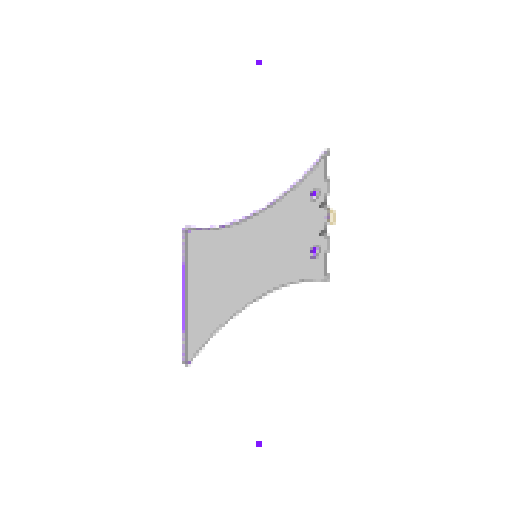
# Autodesk Inventor part: грань тела
Saved by Autodesk Inventor 2023.2 (Build 272271030, 271C)
## iProperties
Created: 2024-11-21
Part Number: грань тела
Material: Типовые
Document SubType Name: Modeling
Designer: DELL
Density: 1 g/cm^3
Appearance: По умолчанию
Author: DELL
Autodesk Inventor part; units mm, degrees
ref_plane "YZ Plane" through (0, 0, 0) normal (1, 0, 0) x (0, 1, 0)
ref_plane "XZ Plane" through (0, 0, 0) normal (0, 1, 0) x (-1, 0, 0)
ref_plane "РабПлоскость1" through (0, 0, -4) normal (0, 0, 1) x (1, 0, 0)
sketch "Эскиз10" plane through (0, 0, 0) normal (1, 0, 0) x (0, 1, 0)
  line L0 (-120, -3.999984) -> (120, -3.999996) construction
  line L1 (120, -3.999996) -> (120, 276.000004) construction
  line L2 (110.388959, 276.000004) -> (-110.388959, 276.000004)
  line L3 (-120, 276.000004) -> (-120, -3.999984) construction
  line L4 (-110, -3.999985) -> (110, -3.999996)
  arc A0 (-110, -3.999985) -> (-114.536812, 268.208047) centre (-321.93085, 128.609648) ccw
  arc A1 (114.536839, 268.208035) -> (110, -3.999996) centre (321.930876, 128.609584) ccw
  arc A2 (114.536839, 268.208035) -> (110.388959, 276.000004) centre (110.388986, 270.999993) ccw
  arc A3 (-110.388959, 276.000004) -> (-114.536812, 268.208047) centre (-110.388931, 271.000015) ccw
  ellipse E0 centre (-0.000042, -3.999995) end of major axis (-110.000042, -3.999985) minor radius 0.000001 (-77.388201, -3.999987) -> (77.387813, -4.000003) ccw
  point P0 (0, 0)
  point P1 (0, -3.999996)
  dimension "d55" = 5
  dimension "d50" = 240
  dimension "d51" = 280
  dimension "d52" = 220
  dimension "d53" = 250
  dimension "d54" = 250
  constraints: 10 end point, 6 point on circle, 4 horizontal, 2 centre point, 2 midpoint, 2 parallel, 2 point on line, 1 perpendicular, 12 other
  measures "d50" distance of L3.start L1.end
  measures "d51" distance of L1.end L0.end
  measures "d52" distance of L4.start L4.end
  measures "d53" radius of A0
  measures "d54" radius of A1
extrude "Выдавливание6" add sketch "Эскиз10" along normal mid plane 4
sketch "Эскиз12" plane through (2, 0, 0) normal (1, 0, 0) x (0, 0, -1)
  line L0 (4.106727, -100.959277) -> (0, -100.959277)
  line L1 (0, -100.959277) -> (0, -60.959277)
  line L2 (0, -60.959277) -> (3.999996, -60.959277)
  line L3 (3.999996, 110) -> (3.999996, -110)
  line L4 (3.999996, -110) -> (3.999996, 110)
  line L5 (3.999996, -35.959277) -> (0, -35.959277)
  line L6 (0, -35.959277) -> (0, -12.5)
  line L7 (0, -12.5) -> (3.999996, -12.5)
  line L8 (3.999996, 12.5) -> (0, 12.5)
  line L9 (0, 12.5) -> (0, 35.500352)
  line L10 (0, 35.500352) -> (3.999996, 35.500352)
  line L11 (3.999996, 60.500352) -> (0, 60.500352)
  line L12 (0, 60.500352) -> (0, 100.500352)
  line L13 (0, 100.500352) -> (3.999996, 100.500352)
  point P0 (0, 0)
  point P1 (3.999996, 12.5)
  point P2 (3.999996, 35.500352)
  point P3 (3.999996, -35.959277)
  point P4 (3.999996, -12.5)
  point P5 (3.999996, -100.959277)
  constraints: 24 end point, 10 perpendicular, 7 point on line, 2 horizontal, 8 other
extrude "Выдавливание7" cut sketch "Эскиз12" against normal blind 4
sketch "Эскиз13" plane through (2, 0, 0) normal (1, 0, 0) x (0, 0, -1)
  line L0 (-14.999956, -22.654638) -> (-14.999956, -25.804638)
  line L1 (0, -25.768292) -> (0, -22.690984)
  line L2 (0, -35.959277) -> (0, -12.5)
  line L3 (-6.160767, -27.015984) -> (-8.460767, -27.015984)
  line L4 (-8.460767, -21.515984) -> (-6.160767, -21.515984)
  line L5 (-14.999956, -24.229638) -> (0, -24.229638) construction
  line L6 (0, -12.5) -> (0, -35.959277)
  line L7 (-8.460767, -27.015984) -> (-8.460767, -25.804638)
  line L8 (-8.460767, -22.654638) -> (-8.460767, -21.515984)
  line L9 (-14.999956, -25.804638) -> (-8.460767, -25.804638)
  line L10 (-6.160767, -25.768292) -> (0, -25.768292)
  line L11 (-6.160767, -21.515984) -> (-6.160767, -22.690984)
  line L12 (-6.160767, -25.768292) -> (-6.160767, -27.015984)
  line L13 (0, -22.690984) -> (-6.160767, -22.690984)
  line L14 (-8.460767, -22.654638) -> (-14.999956, -22.654638)
  line L15 (0, 12.5) -> (0, 35.500352)
  line L16 (0, 18.744943) -> (0, 30.612365)
  line L17 (0, 22.425176) -> (0, 25.575176)
  line L18 (-15, 25.575176) -> (-15, 22.425176)
  line L19 (-8.65, 21.250176) -> (-6.35, 21.250176)
  line L20 (-6.35, 26.750176) -> (-8.65, 26.750176)
  line L21 (-15, 24.000176) -> (0, 24.000176) construction
  line L22 (-8.65, 26.750176) -> (-8.65, 25.575176)
  line L23 (-8.65, 22.425176) -> (-8.65, 21.250176)
  line L24 (-15, 22.425176) -> (-8.65, 22.425176)
  line L25 (-6.35, 22.425176) -> (0, 22.425176)
  line L26 (-6.35, 21.250176) -> (-6.35, 22.425176)
  line L27 (-6.35, 25.575176) -> (-6.35, 26.750176)
  line L28 (0, 25.575176) -> (-6.35, 25.575176)
  line L29 (-8.65, 25.575176) -> (-15, 25.575176)
  circle A0 centre (-23.156324, -48.459277) radius 9
  line L30 (3.999996, -35.959277) -> (3.999996, -60.959277)
  line L31 (3.999996, -48.459277) -> (-57.580157, -48.459277) construction
  line L32 (3.999996, 35.500352) -> (3.999996, 60.500352)
  line L33 (0, 0) -> (-64.518783, 0) construction
  circle A1 centre (-23.156324, 48.459277) radius 9
  dimension "d60" = 15
  dimension "d61" = 3.15
  dimension "d62" = 2.3
  dimension "d63" = 5.5
  dimension "d64" = 6.35
  dimension "d70" = 15
  dimension "d71" = 3.15
  dimension "d72" = 2.3
  dimension "d73" = 5.5
  dimension "d77" = 18
  constraints: 58 end point, 20 parallel, 10 perpendicular, 9 midpoint, 8 horizontal, 3 point on line, 2 centre point, 1 symmetric about line, 1 other
  measures "d60" distance of L1.start L0.end
  measures "d61" distance of L0.end L0.start
  measures "d62" distance of L4.start L4.end
  measures "d63" distance of L3.end L4.start
  measures "d64" distance of point (0, -24.23) L11.end
  measures "d70" distance of L18.start L17.end
  measures "d71" distance of L17.end L17.start
  measures "d72" distance of L20.end L20.start
  measures "d73" distance of L20.start L19.end
  measures "d77" diameter of A0
extrude "Выдавливание8" cut sketch "Эскиз13" against normal blind 4
sketch "Эскиз15" plane through (-2, 0, 0) normal (-1, 0, 0) x (0, 0, 1)
  line L0 (0, -22.690984) -> (6.160767, -22.690984) construction
  line L1 (6.160767, -22.690984) -> (6.160767, -21.515984) construction
  line L2 (6.160767, -21.515984) -> (8.460767, -21.515984) construction
  line L3 (8.460767, -21.515984) -> (8.460767, -22.654638) construction
  line L4 (8.460767, -22.654638) -> (14.999956, -22.654638) construction
  line L5 (14.999956, -22.654638) -> (14.999956, -25.804638) construction
  line L6 (14.999956, -25.804638) -> (8.460767, -25.804638) construction
  line L7 (8.460767, -25.804638) -> (8.460767, -27.015984) construction
  line L8 (8.460767, -27.015984) -> (6.160767, -27.015984) construction
  line L9 (6.160767, -27.015984) -> (6.160767, -25.768292) construction
  line L10 (6.160767, -25.768292) -> (0, -25.768292) construction
  line L11 (0, -25.768292) -> (0, -35.959277) construction
  line L12 (0, -35.959277) -> (-3.999996, -35.959277) construction
  line L13 (-3.999996, -35.959277) -> (-3.999996, -60.959277) construction
  line L14 (-3.999996, -60.959277) -> (0, -60.959277) construction
  line L15 (0, -60.959277) -> (0, -100.959277) construction
  line L16 (0, -100.959277) -> (-3.999996, -100.959277) construction
  line L17 (-3.999996, -100.959277) -> (-3.999996, -110) construction
  arc A0 (268.208035, -114.536839) -> (-3.999996, -110) centre (128.609616, -321.930863) ccw construction
  arc A1 (268.208035, -114.536839) -> (276.000004, -110.388959) centre (271.000004, -110.388959) ccw construction
  line L18 (276.000004, -110.388959) -> (276.000004, 110.388959) construction
  arc A2 (276.000004, 110.388959) -> (268.208035, 114.536839) centre (271.000004, 110.388959) ccw construction
  arc A3 (-3.999996, 110) -> (268.208035, 114.536839) centre (128.609616, 321.930863) ccw construction
  line L19 (-3.999996, 110) -> (-3.999996, 100.500352) construction
  line L20 (-3.999996, 100.500352) -> (0, 100.500352) construction
  line L21 (0, 100.500352) -> (0, 60.500352) construction
  line L22 (0, 60.500352) -> (-3.999996, 60.500352) construction
  line L23 (-3.999996, 60.500352) -> (-3.999996, 35.500352) construction
  line L24 (-3.999996, 35.500352) -> (0, 35.500352) construction
  line L25 (0, 35.500352) -> (0, 25.575176) construction
  line L26 (0, 25.575176) -> (6.35, 25.575176) construction
  line L27 (6.35, 25.575176) -> (6.35, 26.750176) construction
  line L28 (6.35, 26.750176) -> (8.65, 26.750176) construction
  line L29 (8.65, 26.750176) -> (8.65, 25.575176) construction
  line L30 (8.65, 25.575176) -> (15, 25.575176) construction
  line L31 (15, 25.575176) -> (15, 22.425176) construction
  line L32 (15, 22.425176) -> (8.65, 22.425176) construction
  line L33 (8.65, 22.425176) -> (8.65, 21.250176) construction
  line L34 (8.65, 21.250176) -> (6.35, 21.250176) construction
  line L35 (6.35, 21.250176) -> (6.35, 22.425176) construction
  line L36 (6.35, 22.425176) -> (0, 22.425176) construction
  line L37 (0, 22.425176) -> (0, 12.5) construction
  line L38 (0, 12.5) -> (-3.999996, 12.5) construction
  line L39 (-3.999996, 12.5) -> (-3.999996, -12.5) construction
  line L40 (-3.999996, -12.5) -> (0, -12.5) construction
  line L41 (0, -12.5) -> (0, -22.690984) construction
  circle A4 centre (23.156324, -48.459277) radius 9 construction
  circle A5 centre (23.156324, 48.459277) radius 9 construction
  line L42 (-0.000003, 57.000157) -> (-0.000003, 61.000157) construction
  line L43 (-0.000003, 61.000157) -> (275.999997, 61.000184) construction
  line L44 (275.999997, 61.000184) -> (275.999997, 57.000184) construction
  line L45 (275.999997, 57.000184) -> (-0.000003, 57.000157) construction
  line L46 (-0.000003, -61.229615) -> (-0.000003, -57.229615) construction
  line L47 (-0.000003, -57.229615) -> (275.999997, -57.229643) construction
  line L48 (275.999997, -57.229643) -> (275.999997, -61.229643) construction
  line L49 (275.999997, -61.229643) -> (-0.000003, -61.229615) construction
  line L50 (275.999997, 57.000184) -> (-0.000003, 57.000184)
  line L51 (-0.000003, 57.000184) -> (-0.000003, -57.229615)
  line L52 (-0.000003, -57.229615) -> (275.999997, -57.229615)
  line L53 (275.999997, -57.229615) -> (275.999997, 57.000184)
  point P0 (0, 0)
  constraints: 108 end point, 11 centre point, 8 point on circle, 2 parallel, 1 horizontal, 1 perpendicular
